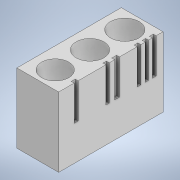
# Autodesk Inventor part: TEST
Saved by Autodesk Inventor 2021 (Build 250183000, 183)
## iProperties
Created: 2022-08-14
Part Number: TEST
Material: Ogólny
Document SubType Name: Modeling
Designer: MicnedSQ
Density: 1 g/cm^3
Appearance: Domyślna
Author: MicnedSQ
Autodesk Inventor part; units mm, degrees
ref_plane "YZ Plane" through (0, 0, 0) normal (1, 0, 0) x (0, 1, 0)
ref_plane "XZ Plane" through (0, 0, 0) normal (0, 1, 0) x (-1, 0, 0)
ref_plane "XY Plane" through (0, 0, 0) normal (0, 0, 1) x (1, 0, 0)
sketch "Szkic1" plane through (0, 0, 0) normal (0, 1, 0) x (-1, 0, 0)
  line L0 (3, 7.5) -> (-3, 7.5)
  line L1 (-3, 7.5) -> (-3, -7.5)
  line L2 (-3, -7.5) -> (3, -7.5)
  line L3 (3, -7.5) -> (3, 7.5)
  point P0 (0, 0)
  point P1 (0, -7.5)
  point P2 (3, 0)
  dimension "d0" = 6
  dimension "d1" = 15
  constraints: 8 end point, 2 midpoint, 2 parallel, 1 horizontal, 1 horizontal alignment, 1 perpendicular, 1 vertical alignment
  measures "d0" distance of L2.end L1.end
  measures "d1" distance of L1.end L0.end
extrude "Wyciągnięcie proste1" add sketch "Szkic1" along normal blind 10
sketch "Szkic2" plane through (0, 10, 0) normal (0, 1, 0) x (1, 0, 0)
  circle A0 centre (0, -5) radius 1.95
  circle A1 centre (0, 0) radius 2
  circle A2 centre (0, 5) radius 2.05
  dimension "d4" = 3.9
  dimension "d5" = 4
  dimension "d6" = 4.1
  dimension "d7" = 5
  dimension "d8" = 5
  constraints: 3 centre point, 1 coincident
  measures "d4" diameter of A0
  measures "d5" diameter of A1
  measures "d6" diameter of A2
  measures "d7" distance of point (0, 0) A0.centre
  measures "d8" distance of A2.centre point (0, 0)
extrude "Wyciągnięcie proste2" cut sketch "Szkic2" against normal blind 9
sketch "Szkic3" plane through (0, 10, 0) normal (0, 1, 0) x (1, 0, 0)
  line L0 (3, -7.5) -> (3, 7.5) projected
  line L1 (3, -5.2848) -> (2.5823, -5.2848)
  line L2 (2.5823, -5.2848) -> (2.5823, -4.7242)
  line L3 (2.5823, -4.7242) -> (3, -4.7242)
  line L4 (3, -4.7242) -> (3, -5.2848)
  line L5 (3, -0.7206) -> (2.5823, -0.7206)
  line L6 (2.5823, -0.7206) -> (2.5823, -0.2402)
  line L7 (2.5823, -0.2402) -> (3, -0.2402)
  line L8 (3, -0.2402) -> (3, -0.7206)
  line L9 (3, 0.5405) -> (2.5823, 0.5405)
  line L10 (2.5823, 0.5405) -> (2.5823, 1.2211)
  line L11 (2.5823, 1.2211) -> (3, 1.2211)
  line L12 (3, 1.2211) -> (3, 0.5405)
  line L13 (3, 3.7634) -> (2.5823, 3.7634)
  line L14 (2.5823, 3.7634) -> (2.5823, 4.3039)
  line L15 (2.5823, 4.3039) -> (3, 4.3039)
  line L16 (3, 4.3039) -> (3, 3.7634)
  line L17 (3, 4.9244) -> (2.5823, 4.9244)
  line L18 (2.5823, 4.9244) -> (2.5823, 5.4049)
  line L19 (2.5823, 5.4049) -> (3, 5.4049)
  line L20 (3, 5.4049) -> (3, 4.9244)
  line L21 (3, 5.9453) -> (2.5823, 5.9453)
  line L22 (2.5823, 5.9453) -> (2.5823, 6.4858)
  line L23 (2.5823, 6.4858) -> (3, 6.4858)
  line L24 (3, 6.4858) -> (3, 5.9453)
  point P0 (0, 0)
  constraints: 48 end point, 12 parallel, 11 point on line, 6 horizontal, 6 perpendicular
extrude "Wyciągnięcie proste3" cut sketch "Szkic3" against normal blind 5
